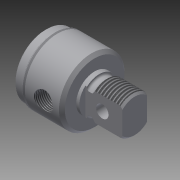
# Autodesk Inventor part: 12P0000_rear_head
Saved by Autodesk Inventor 2014 SP2 (Build 180246200, 246)
## iProperties
Created: 2019-01-29
Part Number: 12P0000_rear_head
Material: Generic
Catalog Web Link: www.cadenas.de
Description: Rear Head-Original Line - Standard Air Cylinders
Vendor: BIMBA
Document SubType Name: Modeling
Designer: psadmin
Manufacturer: BIMBA
Mass: 20.1617 g
Surface Area: 74.4239 cm^2
Volume: 20.1617 cm^3
Density: 1 g/cm^3
Appearance: PSOLRGB-211-211-211
Category: PARTsolutions
Company: BIMBA
Title: 12P0000_rear_head
Author: Cadenas PARTsolutions
Comments: Original Line - Standard Air Cylinders
PSOL_IDENT_0: {$CADENAS_DATA\23d-libs\bimba\bimba\bimba_imperial\bimba_full_line\original_line_cylinders\standard_
PSOL_IDENT_1: air_cylinders\rear_head.prj},239 {VTYP=3D},{NB=12P0000_rear_head},{LINA=12P0000_rear_head},{NN=Rear
PSOL_IDENT_2: Head},{DATE=21.03.2018 14:31:21},{GEOMDATE=30.06.2014 06:34:00},{VERSION=},{LINEID=70},{WBVAR=MNT,AC
PSOL_IDENT_3: TING,DER,Q,T1,T2,T3,T4,TRIM,Y,K,MB,CUSH,FBON},{WBNUMERIC=TRIM,MB,CUSH}  {NB=12P0000_rear_head},{LINA=
PSOL_IDENT_4: 12P0000_rear_head},{KT=DUMMY},{PN=12P0000},{BORE=1.25000},{BOREPN=12},{MNT=P},{MNTALG='' , 'Front No
PSOL_IDENT_5: se' , 'P' , 'Rear Pivot' , 'LS' , 'Built-in Valve LS' , 'DX' , 'Double End'},{ACTING=},{ACTINGALG= ''
PSOL_IDENT_6: , 'Single Acting' , 'R' , 'Reverse/Double Acting' },{DER=},{DERALG= '' , 'Standard' },{Q=},{T1=},{T
PSOL_IDENT_7: 2=},{T3=},{T4=},{TRIM=0},{Y=},{K=},{KALG= '', 'without K', 'K', 'with K' },{MB=0},{A1=1.8120},{A1N=0
PSOL_IDENT_8: .6880},{A1P=1.8120},{A1B=0.0000},{A1S=1.1250},{A2=0.25},{A2N=0.2500},{A3=0.0400},{D1=1.3265},{D1N=1.
PSOL_IDENT_9: 3265},{D1P=1.3265},{D1B=0.0000},{D2=1.2615},{C1=0.0300},{C2=0.0300},{NDM=0.4050},{TAB=NPT},{NDMDP=0.
PSOL_IDENT_10: 2730},{D3=0.3440},{A4=0.2500},{A5=0.8705},{D4=0.8750},{A6=0.3120},{A7=0.7500},{A8=0.0000},{D5=0.0000
PSOL_IDENT_11: },{D6=0.5000},{A9=0.8120},{NDM2=0.7500},{TAB2=UNF},{C11=0.0300},{C22=0.0000},{C33=0.0000},{C44=0.060
PSOL_IDENT_12: 0},{A10=0.5000},{A11=0.0000},{NDM3=0.4050},{NDM3N=0.4050},{NDM3B=0.0000},{TAB3=NPT},{TAB3N=NPT},{TAB
PSOL_IDENT_13: 3B=-},{A12=0.625},{A12N=0.6250},{A12B=0.0000},{A13=1.4060},{D7=0.2520},{D8=0.7475},{A14=0.0940},{A15=
PSOL_IDENT_14: 0.0965},{D9=0.6535},{R1=0.0400},{X1=0.8750},{X2=0.3120},{CX=0.0000},{CC=1.0620},{CON=1},{S1=0.0000},
PSOL_IDENT_15: {DB=0.0000},{X1B=0.0000},{X2B=0.0000},{A8B=0.0000},{A9B=0.0000},{MODEL=1},{NDM4=0.0000},{TAB4=-},{ND
PSOL_IDENT_16: M4DP=0.0000},{BC=0.0000},{B1=0.0000},{B2=0.0000},{B3=0.0000},{ON=0},{ON2=1},{G1=0.3750},{G2=0.8120},
PSOL_IDENT_17: {G3=0.8130},{G4=0.7475},{GD=0.2520},{G5=1.0000},{G6=0.5000},{RON=0},{H1=1.3265},{H2=0.0000},{H3=0.00
PSOL_IDENT_18: 00},{H4=0.0310},{H5=0.9420},{H6=0.5000},{F=0.0000},{PNUT=1.0940},{CUSH=0},{CC11=0.000},{CC111=0.0000
PSOL_IDENT_19: },{CC22=0.0000},{CC33=0.0000},{CC44=0.0000},{CC55=0.0000},{CD1=0.0000},{CD2=0.0000},{CD3=0.0000},{CN
PSOL_IDENT_20: DM3=0.0000},{CTAB3=0.0000},{OLEN=1.4060},{OD=0.3765},{STDIS=0.3178},{STDIS1=0.3178},{BUSHCON=D-4462}
PSOL_IDENT_21: ,{BUSHL=0.5000},{FBON=0},{LCD=0.0000}
NN: Rear Head
NT: Original Line - Standard Air Cylinders
NB: 12P0000_rear_head
NBSYN: $PN._rear_head
LINA: 12P0000_rear_head
PN: 12P0000
BORE: 1.25
BOREPN: 12
MNT: Rear Pivot
MNTALG: '' , 'Front Nose' , 'P' , 'Rear Pivot' , 'LS' , 'Built-in Valve LS' , 'DX' , 'Double End'
ACTING: Single Acting
DER: Standard
Q: Without Side Ported Rear Head
T1: without T1
T2: without T2
T3: without T3
T4: without T4
TRIM: 0
Y: without Pivot Bushing
K: without K
MB: 0
A1N: 0.688
A1P: 1.812
A1B: 0
A1S: 1.125
A2N: 0.25
A3: 0.04
D1N: 1.3265
D1P: 1.3265
D1B: 0
D2: 1.2615
C1: 0.03
C2: 0.03
TAB: NPT
NDMDP: 0.273
D3: 0.344
A4: 0.25
A5: 0.8705
D4: 0.875
A6: 0.312
A7: 0.75
A8: 0
D5: 0
D6: 0.5
A9: 0.812
NDM2: 0.75
TAB2: UNF
C11: 0.03
C22: 0
C33: 0
C44: 0.06
A10: 0.5
A11: 0
NDM3N: 0.405
NDM3B: 0
TAB3N: NPT
TAB3B: -
A12N: 0.625
A12B: 0
A13: 1.406
D7: 0.252
D8: 0.7475
A14: 0.094
A15: 0.0965
D9: 0.6535
R1: 0.04
X1: 0.875
X2: 0.312
CX: 0
CC: 1.062
S1: 0
DB: 0
X1B: 0
X2B: 0
A8B: 0
A9B: 0
NDM4: 0
TAB4: -
NDM4DP: 0
BC: 0
B1: 0
B2: 0
B3: 0
G1: 0.375
G2: 0.812
G3: 0.813
G4: 0.7475
GD: 0.252
G5: 1
G6: 0.5
H2: 0
H3: 0
F: 0
CUSH: 0
CC111: 0
CC22: 0
CC33: 0
CC44: 0
CC55: 0
CD1: 0
CD2: 0
CD3: 0
CNDM3: 0
CTAB3: 0.0000
OD: 0.3765
STDIS1: 0.3178
BUSHCON: D-4462
BUSHL: 0.5
FBON: 0
LCD: 0
SUPPLIER: BIMBA
ARTICLENO: 12P0000_rear_head
BOMINFO: 12P0000_rear_head
CREATOR: CADENAS GmbH
Autodesk Inventor part; units mm, degrees
sketch "Sketch_18" plane through (0, 0, 0) normal (0, 0, 1) x (1, 0, 0)
  line L0 (25.4, 0) -> (0, 0)
  line L1 (0, 0) -> (0, 15.2591)
  line L2 (0, 15.2591) -> (0.762, 16.021)
  line L3 (0.762, 16.021) -> (4.318, 16.021)
  line L4 (4.318, 16.021) -> (5.334, 15.0051)
  line L5 (5.334, 15.0051) -> (6.35, 15.0051)
  line L6 (6.35, 15.0051) -> (6.35, 16.8466)
  line L7 (6.35, 16.8466) -> (23.876, 16.8466)
  line L8 (23.876, 16.8466) -> (25.4, 15.3226)
  line L9 (25.4, 15.3226) -> (25.4, 0)
  line L10 (25.4, 0) -> (0, 0)
  constraints: 22 end point
revolve "Revolution1" add sketch "Sketch_18" angle 360 about axis through (25.4, 0, 0) along (1, 0, 0)
sketch "Sketch_15" plane through (0, 0, 0) normal (0, 0, 1) x (1, 0, 0)
  line L0 (46.0248, 0) -> (25.4, 0)
  line L1 (25.4, 0) -> (25.4, 9.4932)
  line L2 (25.4, 9.4932) -> (27.7876, 9.4932)
  line L3 (27.7876, 9.4932) -> (27.7876, 9.3155)
  arc A0 (27.7876, 9.3155) -> (28.8036, 8.2995) centre (28.8036, 9.3154) ccw
  line L4 (28.8036, 8.2995) -> (30.2387, 8.2995)
  arc A1 (30.2387, 8.2995) -> (30.873, 8.5218) centre (30.2387, 9.3155) ccw
  line L5 (30.873, 8.5218) -> (30.9571, 8.589)
  line L6 (30.9571, 8.589) -> (31.8931, 9.525)
  line L7 (31.8931, 9.525) -> (45.0888, 9.525)
  line L8 (45.0888, 9.525) -> (46.0248, 8.589)
  line L9 (46.0248, 8.589) -> (46.0248, 0)
  line L10 (46.0248, 0) -> (25.4, 0)
  constraints: 22 end point, 4 point on circle, 2 centre point
revolve "Revolution2" add sketch "Sketch_15" angle 360 about axis through (46.0248, 0, 0) along (1, 0, 0)
thread "Thread1" size "3/4-16 UNF" class "2A" standard "ANSI Unified Screw Threads" full length
sketch "Sketch_9" plane through (46.0248, 0, 0) normal (1, 0, 0) x (0, 0, -1)
  line L0 (-33.6931, -67.3862) -> (33.6931, -67.3862)
  line L1 (33.6931, -67.3862) -> (33.6931, 67.3862)
  line L2 (33.6931, 67.3862) -> (-33.6931, 67.3862)
  line L3 (-33.6931, 67.3862) -> (-33.6931, -67.3862)
  line L4 (-6.35, -33.6931) -> (6.35, -33.6931)
  line L5 (6.35, -33.6931) -> (6.35, 33.6931)
  line L6 (6.35, 33.6931) -> (-6.35, 33.6931)
  line L7 (-6.35, 33.6931) -> (-6.35, -33.6931)
  constraints: 16 end point
extrude "Extrusion1" cut sketch "Sketch_9" against normal blind 19.05
sketch "Sketch4" plane through (0, 0, 0) normal (-1, 0, 0) x (0, 0, 1)
  point P0 (0, 0)
hole "Hole1" at (0, 0, 0) direction (1, 0, 0) diameter 12.7 depth 22.6873 tip angle 120
sketch "Sketch_68" plane through (0, 0, 0) normal (0, 0.9998477, 0.0174524) x (1, 0, 0)
  line L0 (15.875, -16.8465) -> (15.875, 0)
  line L1 (15.875, 0) -> (20.498, 0)
  line L2 (20.498, 0) -> (20.498, -9.9123)
  line L3 (20.498, -9.9123) -> (20.7145, -16.8465)
  line L4 (20.7145, -16.8465) -> (15.875, -16.8465)
  line L5 (15.875, -16.8465) -> (15.875, 0)
  constraints: 12 end point
revolve "Revolution3" cut sketch "Sketch_68" angle 360 about axis through (15.875, -0.294, 16.844) along (0, -0.0174524, 0.9998477)
thread "Thread2" size "1/8" designation "1/8 - 27 NPT" standard "NPT" length 6.9376
sketch "Sketch_20" plane through (0, 0, 0) normal (0, 0, 1) x (1, 0, 0)
  line L0 (7.9248, 0) -> (0, 0)
  line L1 (0, 0) -> (0, 11.1125)
  line L2 (0, 11.1125) -> (7.9248, 11.1125)
  line L3 (7.9248, 11.1125) -> (7.9248, 0)
  line L4 (7.9248, 0) -> (0, 0)
  constraints: 10 end point
revolve "Revolution4" cut sketch "Sketch_20" angle 360 about axis through (7.9248, 0, 0) along (1, 0, 0)
sketch "Sketch_24" plane through (0, 0, 0) normal (0, 0, 1) x (1, 0, 0)
  line L0 (6.35, 0) -> (5.334, 0)
  line L1 (5.0135, 16.8466) -> (5.0135, 16.7624)
  line L2 (5.0135, 16.7624) -> (6.2166, 15.5593)
  arc A0 (6.2166, 15.3797) -> (6.2166, 15.5593) centre (6.1268, 15.4695) ccw
  line L3 (6.2166, 15.3797) -> (5.842, 15.0051)
  line L4 (5.842, 15.0051) -> (5.334, 15.0051)
  line L5 (5.334, 15.0051) -> (5.334, 14.7511)
  line L6 (5.334, 14.7511) -> (6.35, 14.7511)
  line L7 (6.35, 14.7511) -> (6.35, 15.7133)
  line L8 (6.35, 15.7133) -> (5.2167, 16.8466)
  line L9 (5.2167, 16.8466) -> (5.0135, 16.8466)
  constraints: 20 end point, 2 point on circle, 1 centre point
revolve "Revolution5" add sketch "Sketch_24" angle 360 about axis through (6.35, 0, 0) along (1, 0, 0)
sketch "Sketch_43" plane through (0, 0, 0) normal (0, 0, 1) x (1, 0, 0)
  circle A0 centre (35.7124, 0) radius 3.2004
  constraints: 1 centre point
extrude "Extrusion2" cut sketch "Sketch_43" along normal mid plane 19.05
ref_plane "1_XY" through (27.7876, 0, 0) normal (1, 0, 0) x (0, 0, -1)
ref_plane "1_YZ" through (27.7876, 0, 0) normal (0, 0, -1) x (0, 1, 0)
ref_plane "1_ZX" through (27.7876, 0, 0) normal (0, 1, 0) x (1, 0, 0)
ref_plane "c1_XY" through (25.4, 9.4932, 0) normal (0, 0, 1) x (1, 0, 0)
ref_plane "c1_YZ" through (25.4, 9.4932, 0) normal (1, 0, 0) x (0, 1, 0)
ref_plane "c1_ZX" through (25.4, 9.4932, 0) normal (0, 1, 0) x (0, 0, 1)
ref_plane "c2_XY" through (25.4, -9.4932, 0) normal (0, 0, 1) x (1, 0, 0)
ref_plane "c2_YZ" through (25.4, -9.4932, 0) normal (1, 0, 0) x (0, 1, 0)
ref_plane "c2_ZX" through (25.4, -9.4932, 0) normal (0, 1, 0) x (0, 0, 1)
ref_plane "cc1_XY" through (25.4, 0, 0) normal (0, 0, 1) x (1, 0, 0)
ref_plane "cc1_YZ" through (25.4, 0, 0) normal (1, 0, 0) x (0, 1, 0)
ref_plane "cc1_ZX" through (25.4, 0, 0) normal (0, 1, 0) x (0, 0, 1)
ref_plane "cc2_XY" through (27.7876, 0, 0) normal (0, 0, 1) x (1, 0, 0)
ref_plane "cc2_YZ" through (27.7876, 0, 0) normal (1, 0, 0) x (0, 1, 0)
ref_plane "cc2_ZX" through (27.7876, 0, 0) normal (0, 1, 0) x (0, 0, 1)
ref_plane "lovra1_XY" through (39.6748, 0, 0) normal (1, 0, 0) x (0, 0, -1)
ref_plane "lovra1_YZ" through (39.6748, 0, 0) normal (0, 0, -1) x (0, 1, 0)
ref_plane "lovra1_ZX" through (39.6748, 0, 0) normal (0, 1, 0) x (1, 0, 0)
ref_plane "lovra2_XY" through (39.6748, 11.0554, 0) normal (1, 0, 0) x (0, 0, -1)
ref_plane "lovra2_YZ" through (39.6748, 11.0554, 0) normal (0, 0, -1) x (0, 1, 0)
ref_plane "lovra2_ZX" through (39.6748, 11.0554, 0) normal (0, 1, 0) x (1, 0, 0)
ref_plane "lovra21_XY" through (0, 0, 5.2705) normal (1, 0, 0) x (0, 0, -1)
ref_plane "lovra21_YZ" through (0, 0, 5.2705) normal (0, 0, -1) x (0, 1, 0)
ref_plane "lovra21_ZX" through (0, 0, 5.2705) normal (0, 1, 0) x (1, 0, 0)
ref_plane "lovra22_XY" through (0, 0, -5.2705) normal (1, 0, 0) x (0, 0, -1)
ref_plane "lovra22_YZ" through (0, 0, -5.2705) normal (0, 0, -1) x (0, 1, 0)
ref_plane "lovra22_ZX" through (0, 0, -5.2705) normal (0, 1, 0) x (1, 0, 0)
ref_plane "lovra3_XY" through (39.6748, -11.0554, 0) normal (1, 0, 0) x (0, 0, -1)
ref_plane "lovra3_YZ" through (39.6748, -11.0554, 0) normal (0, 0, -1) x (0, 1, 0)
ref_plane "lovra3_ZX" through (39.6748, -11.0554, 0) normal (0, 1, 0) x (1, 0, 0)
ref_plane "olen_XY" through (35.7124, 0, 0) normal (1, 0, 0) x (0, 0, -1)
ref_plane "olen_YZ" through (35.7124, 0, 0) normal (0, 0, -1) x (0, 1, 0)
ref_plane "olen_ZX" through (35.7124, 0, 0) normal (0, 1, 0) x (1, 0, 0)
ref_plane "p1_XY" through (46.0248, 0, 6.35) normal (1, 0, 0) x (0, 0, -1)
ref_plane "p1_YZ" through (46.0248, 0, 6.35) normal (0, 0, -1) x (0, 1, 0)
ref_plane "p1_ZX" through (46.0248, 0, 6.35) normal (0, 1, 0) x (1, 0, 0)
ref_plane "p2_XY" through (46.0248, 0, -6.35) normal (1, 0, 0) x (0, 0, -1)
ref_plane "p2_YZ" through (46.0248, 0, -6.35) normal (0, 0, -1) x (0, 1, 0)
ref_plane "p2_ZX" through (46.0248, 0, -6.35) normal (0, 1, 0) x (1, 0, 0)
ref_plane "port_XY" through (15.875, 0, 0) normal (0, 0, 1) x (1, 0, 0)
ref_plane "port_YZ" through (15.875, 0, 0) normal (1, 0, 0) x (0, 1, 0)
ref_plane "port_ZX" through (15.875, 0, 0) normal (0, 1, 0) x (0, 0, 1)
ref_plane "port2_XY" through (46.0248, 0, 0) normal (1, 0, 0) x (0, 0, -1)
ref_plane "port2_YZ" through (46.0248, 0, 0) normal (0, 0, -1) x (0, 1, 0)
ref_plane "port2_ZX" through (46.0248, 0, 0) normal (0, 1, 0) x (1, 0, 0)
ref_plane "thd1_XY" through (46.0248, 0, 9.525) normal (1, 0, 0) x (0, 0, -1)
ref_plane "thd1_YZ" through (46.0248, 0, 9.525) normal (0, 0, -1) x (0, 1, 0)
ref_plane "thd1_ZX" through (46.0248, 0, 9.525) normal (0, 1, 0) x (1, 0, 0)
ref_plane "thd2_XY" through (46.0248, 0, -9.525) normal (1, 0, 0) x (0, 0, -1)
ref_plane "thd2_YZ" through (46.0248, 0, -9.525) normal (0, 0, -1) x (0, 1, 0)
ref_plane "thd2_ZX" through (46.0248, 0, -9.525) normal (0, 1, 0) x (1, 0, 0)
ref_plane "to_mounting_bracket_XY" through (25.4, 0, 0) normal (1, 0, 0) x (0, 0, -1)
ref_plane "to_mounting_bracket_YZ" through (25.4, 0, 0) normal (0, 0, -1) x (0, 1, 0)
ref_plane "to_mounting_bracket_ZX" through (25.4, 0, 0) normal (0, 1, 0) x (1, 0, 0)
ref_plane "to_nut_XY" through (27.7876, 0, 0) normal (1, 0, 0) x (0, 0, -1)
ref_plane "to_nut_YZ" through (27.7876, 0, 0) normal (0, 0, -1) x (0, 1, 0)
ref_plane "to_nut_ZX" through (27.7876, 0, 0) normal (0, 1, 0) x (1, 0, 0)
ref_plane "to_pin_XY" through (35.7124, 0, 0) normal (0, 0, 1) x (1, 0, 0)
ref_plane "to_pin_YZ" through (35.7124, 0, 0) normal (1, 0, 0) x (0, 1, 0)
ref_plane "to_pin_ZX" through (35.7124, 0, 0) normal (0, 1, 0) x (0, 0, 1)
ref_plane "to_screw_XY" through (15.875, 0, 0) normal (0, 1, 0) x (1, 0, 0)
ref_plane "to_screw_YZ" through (15.875, 0, 0) normal (1, 0, 0) x (0, 0, -1)
ref_plane "to_screw_ZX" through (15.875, 0, 0) normal (0, 0, -1) x (0, 1, 0)
ref_plane "to_tube_XY" through (5.334, 0, 0) normal (1, 0, 0) x (0, 0, -1)
ref_plane "to_tube_YZ" through (5.334, 0, 0) normal (0, 0, -1) x (0, 1, 0)
ref_plane "to_tube_ZX" through (5.334, 0, 0) normal (0, 1, 0) x (1, 0, 0)
body "Solid1"
